Autodesk Inventor part; units mm, degrees
note: some values were not read from the file. Chosen so that the rebuilt part matches the saved one: direction of "Hole2".
(part 19 of 20)
  line L1608 (7.786286, -8.278547) -> (8.03493, -8.252551)
  line L1609 (8.03493, -8.252551) -> (8.035159, -8.252627)
  line L1610 (6.791707, -8.382529) -> (6.77091, -8.183613)
  line L1611 (6.543062, -8.408524) -> (6.791707, -8.382529)
  line L1612 (8.217517, -9.99687) -> (8.035159, -8.252627)
  line L1613 (7.010297, -10.471221) -> (7.274453, -10.443604)
  line L1614 (7.765489, -8.079631) -> (6.77091, -8.183613)
  line L1615 (6.543062, -8.408524) -> (6.740628, -10.298225)
  line L1616 (7.010069, -10.471145) -> (8.004648, -10.367163)
  line L1617 (8.232497, -10.142252) -> (8.03493, -8.252551)
  line L1618 (6.740856, -10.298301) -> (6.989283, -10.272328)
  line L1619 (6.740628, -10.298225) -> (6.740856, -10.298301)
  line L1620 (6.989273, -10.272229) -> (6.740628, -10.298225)
  line L1621 (7.010069, -10.471145) -> (6.989273, -10.272229)
  line L1622 (7.010297, -10.471221) -> (7.010069, -10.471145)
  line L1623 (7.983852, -10.168247) -> (8.004648, -10.367163)
  line L1624 (8.232497, -10.142252) -> (7.983852, -10.168247)
  line L1625 (6.812503, -8.581445) -> (6.968476, -10.073313)
  line L1626 (7.807082, -8.477462) -> (6.812503, -8.581445)
  line L1627 (7.963055, -9.969331) -> (7.807082, -8.477462)
  line L1628 (6.968476, -10.073313) -> (7.963055, -9.969331)
  line L1629 (7.125675, -9.879662) -> (7.006372, -8.738535)
  line L1630 (6.812503, -8.581445) -> (7.006372, -8.738535)
  line L1631 (6.968476, -10.073313) -> (7.125675, -9.879662)
  line L1632 (7.006372, -8.738535) -> (7.650209, -8.671223)
  line L1633 (7.807082, -8.477462) -> (7.650209, -8.671223)
  line L1634 (7.650209, -8.671223) -> (7.769512, -9.812349)
  line L1635 (7.963055, -9.969331) -> (7.769512, -9.812349)
  line L1636 (7.769512, -9.812349) -> (7.125675, -9.879662)
  circle A34 centre (7.360667, -9.014937) radius 0.1
  line L1637 (7.526698, -9.160376) -> (7.493026, -8.838309)
  line L1638 (7.526731, -9.160387) -> (7.526698, -9.160376)
  line L1639 (7.526731, -9.160387) -> (7.493059, -8.83832)
  line L1640 (7.493059, -8.83832) -> (7.493026, -8.838309)
  line L1641 (7.493026, -8.838309) -> (7.194653, -8.869503)
  line L1642 (7.194653, -8.869503) -> (7.228324, -9.191571)
  line L1643 (7.228357, -9.191582) -> (7.228324, -9.191571)
  line L1644 (7.228324, -9.191571) -> (7.526698, -9.160376)
  line L1645 (7.228357, -9.191582) -> (7.526731, -9.160387)
  line L1646 (3.439822, -8.704549) -> (3.439807, -8.9032)
  line L1647 (3.439807, -8.9032) -> (3.689807, -8.903219)
  line L1648 (2.439807, -8.903124) -> (2.439822, -8.704473)
  line L1649 (2.189807, -8.903105) -> (2.439807, -8.903124)
  line L1650 (3.439651, -10.952678) -> (3.689651, -10.952697)
  line L1651 (3.439664, -10.790392) -> (3.439648, -10.989044)
  line L1652 (3.689664, -10.790411) -> (3.439664, -10.790392)
  line L1653 (3.439648, -10.989044) -> (3.439636, -11.151329)
  line L1654 (3.689651, -10.952697) -> (3.689664, -10.790411)
  line L1655 (2.439636, -11.151253) -> (3.439636, -11.151329)
  line L1656 (3.439822, -8.704549) -> (2.439822, -8.704473)
  line L1657 (2.189807, -8.903105) -> (2.189664, -10.790297)
  line L1658 (2.439648, -10.988968) -> (3.439648, -10.989044)
  line L1659 (3.689664, -10.790411) -> (3.689807, -8.903219)
  line L1660 (2.189651, -10.952583) -> (2.439651, -10.952602)
  line L1661 (2.189664, -10.790297) -> (2.189651, -10.952583)
  line L1662 (2.439664, -10.790316) -> (2.189664, -10.790297)
  line L1663 (2.439648, -10.988968) -> (2.439664, -10.790316)
  line L1664 (2.439636, -11.151253) -> (2.439648, -10.988968)
  line L1665 (2.439792, -9.101776) -> (2.439679, -10.591664)
  line L1666 (3.439792, -9.101852) -> (2.439792, -9.101776)
  line L1667 (3.439679, -10.59174) -> (3.439792, -9.101852)
  line L1668 (2.439679, -10.591664) -> (3.439679, -10.59174)
  line L1669 (2.61601, -10.532458) -> (2.616097, -9.392846)
  line L1670 (2.439792, -9.101776) -> (2.616097, -9.392846)
  line L1671 (2.439679, -10.591664) -> (2.61601, -10.532458)
  line L1672 (2.616097, -9.392846) -> (3.263443, -9.392895)
  line L1673 (3.439792, -9.101852) -> (3.263443, -9.392895)
  line L1674 (3.263443, -9.392895) -> (3.263356, -10.532507)
  line L1675 (3.439679, -10.59174) -> (3.263356, -10.532507)
  line L1676 (3.263356, -10.532507) -> (2.61601, -10.532458)
  ellipse E661 centre (2.939748, -9.673551) end of major axis (2.839748, -9.673543) minor radius 0.099326
  ellipse E662 centre (2.939748, -9.679347) end of major axis (2.839748, -9.679339) minor radius 0.099326 (2.839748, -9.679339) -> (3.039748, -9.679355) ccw
  line L1677 (3.039748, -9.673559) -> (3.039748, -9.679355)
  line L1678 (2.839748, -9.673543) -> (2.839748, -9.679339)
  line L1679 (3.089736, -9.840178) -> (3.08976, -9.518539)
  line L1680 (3.089734, -9.863362) -> (3.089736, -9.840178)
  line L1681 (3.08976, -9.518539) -> (2.78976, -9.518516)
  line L1682 (2.78976, -9.518516) -> (2.789736, -9.840155)
  line L1683 (2.789734, -9.863339) -> (2.789736, -9.840155)
  line L1684 (2.789736, -9.840155) -> (3.089736, -9.840178)
  line L1685 (2.789734, -9.863339) -> (3.089734, -9.863362)
  line L1686 (8.477385, -9.966599) -> (8.477243, -9.966545)
  line L1687 (8.477243, -9.966545) -> (8.500438, -10.165195)
  line L1688 (8.500438, -10.165195) -> (8.748751, -10.136202)
  line L1689 (8.748751, -10.136202) -> (8.748892, -10.136257)
  line L1690 (8.969239, -12.023437) -> (8.748892, -10.136257)
  line L1691 (8.716449, -12.254311) -> (8.74412, -12.25108)
  line L1692 (8.477243, -9.966545) -> (8.2173, -9.996896)
  line L1693 (7.274441, -10.443505) -> (7.479218, -12.19734)
  line L1694 (7.750726, -12.366997) -> (8.743978, -12.251025)
  line L1695 (8.969097, -12.023382) -> (8.748751, -10.136202)
  line L1696 (8.7488, -12.049175) -> (8.969239, -12.023437)
  line L1697 (8.74412, -12.25108) -> (8.732832, -12.154407)
  line L1698 (8.720784, -12.052375) -> (8.743978, -12.251025)
  line L1699 (8.969097, -12.023382) -> (8.720784, -12.052375)
  line L1700 (8.720784, -12.052375) -> (8.720925, -12.052429)
  line L1701 (8.743978, -12.251025) -> (8.74412, -12.25108)
  line L1702 (8.969239, -12.023437) -> (8.969097, -12.023382)
  line L1703 (7.479218, -12.19734) -> (7.47936, -12.197394)
  line L1704 (7.727531, -12.168347) -> (7.479218, -12.19734)
  line L1705 (7.750726, -12.366997) -> (7.727531, -12.168347)
  line L1706 (7.750867, -12.367052) -> (7.750726, -12.366997)
  line L1707 (7.530379, -10.479817) -> (7.704337, -11.969696)
  line L1708 (8.523632, -10.363846) -> (7.530379, -10.479817)
  line L1709 (8.69759, -11.853724) -> (8.523632, -10.363846)
  line L1710 (7.704337, -11.969696) -> (8.69759, -11.853724)
  line L1711 (7.859126, -11.774149) -> (7.726067, -10.634545)
  line L1712 (7.530379, -10.479817) -> (7.726067, -10.634545)
  line L1713 (7.704337, -11.969696) -> (7.859126, -11.774149)
  line L1714 (7.726067, -10.634545) -> (8.369045, -10.559471)
  line L1715 (8.523632, -10.363846) -> (8.369045, -10.559471)
  line L1716 (8.369045, -10.559471) -> (8.502104, -11.699075)
  line L1717 (8.69759, -11.853724) -> (8.502104, -11.699075)
  line L1718 (8.502104, -11.699075) -> (7.859126, -11.774149)
  circle A35 centre (8.083686, -10.906656) radius 0.1
  line L1719 (8.251456, -11.050081) -> (8.213902, -10.728443)
  line L1720 (8.251476, -11.050089) -> (8.251456, -11.050081)
  line L1721 (8.251476, -11.050089) -> (8.213922, -10.728451)
  line L1722 (8.213922, -10.728451) -> (8.213902, -10.728443)
  line L1723 (8.213902, -10.728443) -> (7.915926, -10.763235)
  line L1724 (7.915926, -10.763235) -> (7.95348, -11.084873)
  line L1725 (7.953501, -11.08488) -> (7.95348, -11.084873)
  line L1726 (7.95348, -11.084873) -> (8.251456, -11.050081)
  line L1727 (7.953501, -11.08488) -> (8.251476, -11.050089)
  line L1728 (3.440093, -5.140062) -> (3.440078, -5.339171)
  line L1729 (3.440078, -5.339171) -> (3.690078, -5.33919)
  line L1730 (2.440078, -5.339095) -> (2.440093, -5.139986)
  line L1731 (2.190078, -5.339076) -> (2.440078, -5.339095)
  line L1732 (3.440093, -5.140062) -> (2.440093, -5.139986)
  line L1733 (2.190078, -5.339076) -> (2.189941, -7.14516)
  line L1734 (3.689941, -7.145274) -> (3.690078, -5.33919)
  line L1735 (2.440063, -5.538203) -> (2.439956, -6.946265)
  line L1736 (3.440063, -5.538279) -> (2.440063, -5.538203)
  line L1737 (3.439956, -6.946341) -> (3.440063, -5.538279)
  line L1738 (2.616333, -6.288782) -> (2.616369, -5.808082)
  line L1739 (2.440063, -5.538203) -> (2.616369, -5.808082)
  line L1740 (2.616369, -5.808082) -> (3.263715, -5.808131)
  line L1741 (3.440063, -5.538279) -> (3.263715, -5.808131)
  line L1742 (3.263715, -5.808131) -> (3.263679, -6.288832)
  ellipse E663 centre (2.940021, -6.094897) end of major axis (2.840021, -6.09489) minor radius 0.099554
  ellipse E664 centre (2.94002, -6.099613) end of major axis (2.84002, -6.099606) minor radius 0.099554 (2.84002, -6.099606) -> (3.04002, -6.099621) ccw
  line L1743 (3.040021, -6.094905) -> (3.04002, -6.099621)
  line L1744 (2.840021, -6.09489) -> (2.84002, -6.099606)
  line L1745 (3.090008, -6.260814) -> (3.090033, -5.938435)
  line L1746 (3.090007, -6.279679) -> (3.090008, -6.260814)
  line L1747 (3.090033, -5.938435) -> (2.790033, -5.938413)
  line L1748 (2.790033, -5.938413) -> (2.790008, -6.260792)
  line L1749 (2.790007, -6.279657) -> (2.790008, -6.260792)
  line L1750 (2.790008, -6.260792) -> (3.090008, -6.260814)
  line L1751 (2.790007, -6.279657) -> (3.090007, -6.279679)
  line L1752 (7.201687, -6.366416) -> (7.182831, -6.167323)
  line L1753 (7.182831, -6.167323) -> (7.182731, -6.167316)
  line L1754 (7.182731, -6.167316) -> (7.201589, -6.366425)
  line L1755 (7.201589, -6.366425) -> (7.450475, -6.342853)
  line L1756 (7.450475, -6.342853) -> (7.450575, -6.34286)
  line L1757 (6.206044, -6.460713) -> (6.187186, -6.261604)
  line L1758 (5.957157, -6.484285) -> (6.206044, -6.460713)
  line L1759 (7.471423, -6.562983) -> (7.450575, -6.34286)
  line L1760 (7.182731, -6.167316) -> (6.187186, -6.261604)
  line L1761 (5.957157, -6.484285) -> (6.136303, -8.37582)
  line L1762 (6.404047, -8.551357) -> (6.556485, -8.53692)
  line L1763 (7.61644, -8.095214) -> (7.450475, -6.342853)
  line L1764 (6.136303, -8.37582) -> (6.136404, -8.375826)
  line L1765 (6.38519, -8.352248) -> (6.136303, -8.37582)
  line L1766 (6.404047, -8.551357) -> (6.38519, -8.352248)
  line L1767 (6.404147, -8.551364) -> (6.404047, -8.551357)
  line L1768 (6.224901, -6.659822) -> (6.366332, -8.153139)
  line L1769 (7.220446, -6.565534) -> (6.224901, -6.659822)
  line L1770 (7.361877, -8.058852) -> (7.220446, -6.565534)
  line L1771 (6.366332, -8.153139) -> (7.361877, -8.058852)
  line L1772 (6.52532, -7.960977) -> (6.41714, -6.818742)
  line L1773 (6.224901, -6.659822) -> (6.41714, -6.818742)
  line L1774 (6.366332, -8.153139) -> (6.52532, -7.960977)
  line L1775 (6.41714, -6.818742) -> (7.061602, -6.757706)
  line L1776 (7.220446, -6.565534) -> (7.061602, -6.757706)
  line L1777 (7.061602, -6.757706) -> (7.169782, -7.89994)
  line L1778 (7.361877, -8.058852) -> (7.169782, -7.89994)
  line L1779 (7.169782, -7.89994) -> (6.52532, -7.960977)
  circle A36 centre (6.768748, -7.098596) radius 0.1
  line L1780 (6.933349, -7.245643) -> (6.902817, -6.923263)
  line L1781 (6.933364, -7.245644) -> (6.902831, -6.923263)
  line L1782 (6.902817, -6.923263) -> (6.604154, -6.951549)
  line L1783 (6.604154, -6.951549) -> (6.634686, -7.273929)
  line L1784 (6.634686, -7.273929) -> (6.933349, -7.245643)
  ellipse E665 centre (-10.520754, -10.238556) end of major axis (-11.719228, -10.299056) minor radius 0.214474 (-9.764112, -10.035048) -> (-11.697324, -10.33696) ccw
  ellipse E666 centre (-10.510833, -10.435086) end of major axis (-11.509561, -10.485502) minor radius 0.178729 (-9.978797, -10.257642) -> (-11.297119, -10.583852) ccw
  line L1785 (-11.491308, -10.517089) -> (-11.697324, -10.33696)
  ellipse E667 centre (-10.510833, -10.435086) end of major axis (-11.259879, -10.472898) minor radius 0.134046 (-10.235366, -10.296818) -> (-11.050291, -10.554562) ccw
  line L1786 (-11.719228, -10.299056) -> (-11.762061, -9.450552)
  ellipse E668 centre (10.530165, -10.240157) end of major axis (11.72863, -10.300839) minor radius 0.214474 (11.70672, -10.33874) -> (9.773554, -10.036533) ccw
  ellipse E669 centre (10.520214, -10.436685) end of major axis (11.518935, -10.487253) minor radius 0.178729 (11.306477, -10.585571) -> (9.988205, -10.259161) ccw
  line L1787 (11.500677, -10.518837) -> (11.70672, -10.33874)
  ellipse E670 centre (10.520214, -10.436685) end of major axis (11.269255, -10.474611) minor radius 0.134046 (11.059654, -10.556244) -> (10.244768, -10.298376) ccw
  line L1788 (11.72863, -10.300839) -> (11.771592, -9.452341)
  ellipse E671 centre (0.005822, 4.447603) end of major axis (-0.560598, 4.447646) minor radius 0.563895 (0.374763, 4.019735) -> (-0.363184, 4.019791) ccw
  line L1789 (-0.107751, 4.840436) -> (0.290762, 4.741938)
  line L1790 (0.290762, 4.741938) -> (0.404336, 4.349105)
  line L1791 (0.404336, 4.349105) -> (0.142592, 4.078731)
  line L1792 (-0.108974, 4.111214) -> (-0.279118, 4.153268)
  line L1793 (-0.279118, 4.153268) -> (-0.392691, 4.546101)
  line L1794 (-0.392691, 4.546101) -> (-0.107751, 4.840436)
  line L1795 (0.290762, 4.741938) -> (0.290756, 4.652243)
  line L1796 (-0.107758, 4.751181) -> (-0.107751, 4.840436)
  spline S53 degree 3 poles (-11.59262, -40.37168) (-11.587874, -40.372306) (-11.577549, -40.373667) (-11.562894, -40.383311) (-11.548322, -40.397841) (-11.53396, -40.418162) (-11.520082, -40.443816) (-11.501451, -40.486582) (-11.485653, -40.535603) (-11.472041, -40.590104) (-11.458687, -40.654476) (-11.445359, -40.742787) (-11.436003, -40.854008) (-11.432673, -40.968592) (-11.436021, -41.083176) (-11.445393, -41.194396) (-11.458735, -41.282705) (-11.472098, -41.347075) (-11.485719, -41.401574) (-11.501524, -41.450592) (-11.520162, -41.493356) (-11.534044, -41.519008) (-11.548409, -41.539326) (-11.562983, -41.553853) (-11.577639, -41.563495) (-11.587965, -41.564855) (-11.592711, -41.56548) knots 0 0 0 0 0.01106677 0.02407754 0.03992786 0.05913986 0.0819337 0.10802006 0.16805875 0.20201508 0.23929564 0.3216678 0.41056278 0.5 0.58943722 0.6783322 0.76070436 0.79798492 0.83194125 0.89197994 0.9180663 0.94086014 0.96007214 0.97592246 0.98893323 1 1 1 1
  spline S54 degree 3 poles (-11.592711, -41.56548) (-11.597373, -41.56487) (-11.60739, -41.56356) (-11.621305, -41.553879) (-11.634543, -41.539274) (-11.647072, -41.518918) (-11.658696, -41.49325) (-11.673818, -41.450356) (-11.685905, -41.401361) (-11.695951, -41.34698) (-11.705594, -41.28252) (-11.714843, -41.194166) (-11.721147, -41.083055) (-11.723326, -40.96857) (-11.72113, -40.854086) (-11.714809, -40.742975) (-11.705546, -40.654623) (-11.695894, -40.590164) (-11.68584, -40.535785) (-11.673744, -40.486792) (-11.658616, -40.4439) (-11.646989, -40.418234) (-11.634456, -40.39788) (-11.621216, -40.383277) (-11.607299, -40.373599) (-11.597282, -40.37229) (-11.59262, -40.37168) knots 0 0 0 0 0.01099744 0.02362844 0.03895388 0.0576141 0.07990846 0.10559498 0.1652091 0.19914929 0.2365432 0.31951534 0.40940333 0.5 0.59059667 0.68048466 0.7634568 0.80085071 0.8347909 0.89440502 0.92009154 0.9423859 0.96104612 0.97637156 0.98900256 1 1 1 1
  spline S55 degree 3 poles (11.597357, -41.567244) (11.592611, -41.566618) (11.582286, -41.565257) (11.56763, -41.555613) (11.553059, -41.541083) (11.538697, -41.520762) (11.524819, -41.495108) (11.506188, -41.452342) (11.49039, -41.403321) (11.476777, -41.34882) (11.463424, -41.284448) (11.450096, -41.196137) (11.44074, -41.084916) (11.43741, -40.970332) (11.440758, -40.855748) (11.45013, -40.744528) (11.463471, -40.656219) (11.476835, -40.591849) (11.490456, -40.53735) (11.506261, -40.488332) (11.524899, -40.445568) (11.538781, -40.419916) (11.553146, -40.399598) (11.567719, -40.385071) (11.582376, -40.375429) (11.592702, -40.374069) (11.597448, -40.373444) knots 0 0 0 0 0.01106677 0.02407754 0.03992786 0.05913986 0.0819337 0.10802006 0.16805875 0.20201508 0.23929564 0.3216678 0.41056278 0.5 0.58943722 0.6783322 0.76070436 0.79798492 0.83194125 0.89197994 0.9180663 0.94086014 0.96007214 0.97592246 0.98893323 1 1 1 1
  spline S56 degree 3 poles (11.597448, -40.373444) (11.60211, -40.374054) (11.612126, -40.375364) (11.626042, -40.385045) (11.63928, -40.39965) (11.651809, -40.420006) (11.663433, -40.445674) (11.678555, -40.488568) (11.690642, -40.537563) (11.700688, -40.591944) (11.71033, -40.656404) (11.71958, -40.744758) (11.725884, -40.855869) (11.728063, -40.970354) (11.725866, -41.084838) (11.719545, -41.195949) (11.710283, -41.284301) (11.700631, -41.34876) (11.690576, -41.403139) (11.678481, -41.452132) (11.663353, -41.495024) (11.651725, -41.52069) (11.639193, -41.541044) (11.625953, -41.555647) (11.612036, -41.565325) (11.602019, -41.566634) (11.597357, -41.567244) knots 0 0 0 0 0.01099744 0.02362844 0.03895388 0.0576141 0.07990846 0.10559498 0.1652091 0.19914929 0.2365432 0.31951534 0.40940333 0.5 0.59059667 0.68048466 0.7634568 0.80085071 0.8347909 0.89440502 0.92009154 0.9423859 0.96104612 0.97637156 0.98900256 1 1 1 1
  line L1797 (-4.211059, -43.377142) -> (-4.211066, -43.469142)
  line L1798 (-9.152053, -43.468766) -> (-9.152007, -42.868766)
  line L1799 (-4.211066, -43.469142) -> (-9.152053, -43.468766)
  line L1800 (4.215423, -43.469782) -> (4.21543, -43.377782)
  line L1801 (9.156409, -43.470158) -> (4.215423, -43.469782)
  line L1802 (9.156455, -42.870158) -> (9.156409, -43.470158)
  line L1803 (-3.997776, -42.869158) -> (-9.152007, -42.868766)
  line L1804 (9.156455, -42.870158) -> (4.002224, -42.869766)
  line L1805 (11.952178, -43.470371) -> (9.156409, -43.470158)
  line L1806 (-9.152053, -43.468766) -> (-11.947822, -43.468553)
  line L1807 (4.002559, -38.469766) -> (11.952559, -38.470371)
  line L1808 (-11.947441, -38.468553) -> (-3.997441, -38.469158)
  line L1809 (-11.947822, -43.468553) -> (-11.947441, -38.468553)
  line L1810 (11.952178, -43.470371) -> (11.952559, -38.470371)
  line L1811 (4.215423, -43.469782) -> (3.905563, -43.469759)
  line L1812 (3.905563, -43.469759) -> (3.90557, -43.377759)
  line L1813 (3.905563, -43.469759) -> (-4.211066, -43.469142)
  line L1814 (-9.079045, -28.468771) -> (-3.321818, -28.469209)
  line L1815 (3.328456, -28.469715) -> (9.085683, -28.470153)
  line L1816 (10.653551, -28.470272) -> (11.216615, -28.470315)
  line L1817 (-11.209977, -28.468609) -> (-10.646913, -28.468652)
  line L1818 (11.215854, -38.470315) -> (11.216615, -28.470315)
  line L1819 (-11.209977, -28.468609) -> (-11.210737, -38.468609)
  spline S57 degree 3 poles (-8.765036, -35.867834) (-8.764769, -35.757599) (-8.761349, -35.533673) (-8.743222, -35.201238) (-8.713054, -34.928041) (-8.679705, -34.738723) (-8.645211, -34.64651) (-8.621798, -34.584045) (-8.572571, -34.581581) (-8.544972, -34.621627) (-8.510145, -34.702211) (-8.473031, -34.888434) (-8.44157, -35.161759) (-8.42366, -35.493232) (-8.419288, -35.826558) (-8.426873, -36.159477) (-8.446891, -36.493359) (-8.478808, -36.765397) (-8.514628, -36.955068) (-8.547047, -37.046324) (-8.57088, -37.112013) (-8.620232, -37.11221) (-8.646582, -37.070723) (-8.67735, -36.990083) (-8.714426, -36.804321) (-8.743636, -36.531889) (-8.761168, -36.199722) (-8.765301, -35.977117) (-8.765036, -35.867834) knots 0 0 0 0 0.06370705 0.12949472 0.19191208 0.22368799 0.2382902 0.25135028 0.25660425 0.26301775 0.27714857 0.30853838 0.37103998 0.43687849 0.50002298 0.56369496 0.62938323 0.69283553 0.72316052 0.73857311 0.75180992 0.75696152 0.7632602 0.77795176 0.80804313 0.87131401 0.93684349 1 1 1 1
  spline S58 degree 3 poles (-10.961204, -35.786075) (-10.960572, -35.563356) (-10.950183, -35.239504) (-10.950113, -34.843101) (-10.912349, -34.685004) (-10.92157, -34.591209) (-10.884933, -34.581169) (-10.874211, -34.661615) (-10.855678, -34.748938) (-10.840659, -34.969236) (-10.82721, -35.239057) (-10.81991, -35.572905) (-10.815873, -36.019318) (-10.831573, -36.452197) (-10.835133, -36.849308) (-10.874852, -37.008191) (-10.865551, -37.102751) (-10.902892, -37.113246) (-10.911506, -37.030807) (-10.929507, -36.943774) (-10.941719, -36.722668) (-10.957752, -36.345334) (-10.961836, -36.009053) (-10.961204, -35.786075) knots 0 0 0 0 0.13139199 0.19506211 0.22486648 0.236537 0.23877104 0.24363774 0.27264718 0.30298792 0.36807806 0.43503205 0.49911295 0.63103815 0.69471519 0.72474683 0.73665002 0.73889428 0.74387281 0.77307947 0.80345172 0.86845517 1 1 1 1
  spline S59 degree 3 poles (8.426688, -35.787549) (8.427022, -35.677218) (8.430095, -35.452601) (8.451958, -35.123731) (8.481432, -34.843077) (8.528867, -34.676495) (8.564967, -34.584637) (8.613971, -34.583373) (8.657301, -34.645523) (8.687787, -34.756551) (8.724589, -34.96873) (8.751757, -35.244846) (8.768138, -35.576173) (8.772309, -35.909457) (8.765265, -36.242834) (8.745686, -36.572028) (8.715121, -36.851569) (8.671368, -37.019168) (8.639129, -37.111061) (8.589647, -37.114782) (8.545979, -37.049233) (8.518251, -36.940131) (8.476898, -36.727728) (8.449753, -36.452792) (8.430699, -36.119621) (8.426358, -35.896767) (8.426688, -35.787549) knots 0 0 0 0 0.06377364 0.12947571 0.19191728 0.22251596 0.23572674 0.24098241 0.24712107 0.27642984 0.3084167 0.37100213 0.43691035 0.50001881 0.5637377 0.62924964 0.69193924 0.72212339 0.73538665 0.74053978 0.7469427 0.77702751 0.80721947 0.87118814 0.93686953 1 1 1 1
  line L1820 (9.085683, -28.470153) -> (10.653551, -28.470272)
  line L1821 (-10.646913, -28.468652) -> (-9.079045, -28.468771)
  spline S60 degree 3 poles (10.823981, -35.869324) (10.82469, -35.64542) (10.826632, -35.311386) (10.851011, -34.9324) (10.859679, -34.739412) (10.883274, -34.654106) (10.87675, -34.588309) (10.91413, -34.584971) (10.917546, -34.630294) (10.937011, -34.702577) (10.945793, -34.894313) (10.960284, -35.162958) (10.965785, -35.495284) (10.96758, -35.940764) (10.964119, -36.386459) (10.943062, -36.763358) (10.935643, -36.958091) (10.914064, -37.040444) (10.921591, -37.112085) (10.883957, -37.111227) (10.880857, -37.065642) (10.861355, -36.992736) (10.84984, -36.80192) (10.827243, -36.425919) (10.823277, -36.091835) (10.823981, -35.869324) knots 0 0 0 0 0.13209168 0.19547472 0.22735918 0.24158397 0.25296859 0.25518606 0.26025608 0.27356013 0.30485536 0.36824052 0.43535326 0.4998067 0.63172546 0.69607433 0.72644443 0.74148548 0.75299654 0.75519516 0.76033444 0.77439415 0.80449955 0.86873005 1 1 1 1
  line L1822 (4.003131, -30.939766) -> (2.003688, -23.619614)
  line L1823 (-1.996312, -23.61931) -> (-3.996869, -30.939158)
  line L1824 (4.002263, -42.361766) -> (4.003131, -30.939766)
  line L1825 (-3.997737, -42.361158) -> (-3.996869, -30.939158)
  line L1826 (2.003688, -23.619614) -> (-1.996312, -23.61931)
  line L1827 (4.002263, -42.361766) -> (4.002185, -43.377766)
  line L1828 (-3.997737, -42.361158) -> (-3.997815, -43.377158)
  line L1829 (4.002185, -43.377766) -> (-3.997815, -43.377158)
  line L1830 (-8.122783, -43.376844) -> (-8.297643, -43.376831)
  line L1831 (-8.122744, -42.868844) -> (-8.122783, -43.376844)
  line L1832 (-4.420375, -43.377126) -> (-8.122783, -43.376844)
  line L1833 (-4.420375, -43.377126) -> (-3.997815, -43.377158)
  line L1834 (4.002185, -43.377766) -> (4.424746, -43.377798)
  line L1835 (8.127153, -43.37808) -> (4.424746, -43.377798)
  line L1836 (8.127192, -42.87008) -> (8.127153, -43.37808)
  line L1837 (8.302013, -43.378093) -> (8.127153, -43.37808)
  line L1838 (-8.297604, -42.868831) -> (-8.297643, -43.376831)
  line L1839 (8.302052, -42.870093) -> (8.302013, -43.378093)
  line L1840 (-10.99805, -46.468625) -> (11.00195, -46.470299)
  line L1841 (-11.000559, -79.468625) -> (10.99944, -79.470298)
  line L1842 (-11.000559, -79.468625) -> (-10.99805, -46.468625)
  line L1843 (10.99944, -79.470298) -> (11.00195, -46.470299)
  line L1844 (-9.396535, -46.468747) -> (-9.396307, -43.468747)
  line L1845 (-7.296535, -46.468907) -> (-7.296307, -43.468907)
  line L1846 (-1.04805, -46.469382) -> (-1.047822, -43.469382)
  line L1847 (1.05195, -46.469542) -> (1.052178, -43.469542)
  line L1848 (7.300435, -46.470017) -> (7.300663, -43.470017)
  line L1849 (9.400435, -46.470177) -> (9.400663, -43.470177)
  spline S61 degree 3 poles (-9.494, -108.299265) (-9.352975, -108.712955) (-9.066555, -109.553156) (-8.690144, -110.85923) (-8.369211, -112.235424) (-8.131096, -113.648007) (-7.981225, -115.049157) (-7.905778, -116.397457) (-7.880518, -117.699949) (-7.880477, -118.554616) (-7.880457, -118.976908) knots 0 0 0 0 0.13110718 0.26627767 0.40758133 0.55482273 0.69573025 0.83010398 0.95981582 1.08650249 1.08650249 1.08650249 1.08650249
  spline S62 degree 3 poles (-11.494, -103.994777) (-11.494, -103.994565) (-11.494, -103.993719) (-11.494, -103.991816) (-11.494, -103.988647) (-11.494, -103.984218) (-11.494, -103.978533) (-11.494, -103.971598) (-11.494, -103.963419) (-11.494, -103.954002) (-11.494, -103.94335) (-11.494, -103.931473) (-11.494, -103.918383) (-11.494, -103.904098) (-11.494, -103.888638) (-11.494, -103.872014) (-11.494, -103.85424) (-11.494, -103.842008) (-11.494, -103.835703) knots 0 0 0 0 0.00398745 0.01595749 0.03589091 0.06374884 0.09949715 0.14310174 0.1945285 0.2537433 0.32071204 0.39540061 0.47774624 0.56757484 0.66479437 0.76932497 0.8810868 1 1 1 1
  spline S63 degree 3 poles (-11.494, -103.835703) (-11.340511, -104.219325) (-11.035906, -104.980636) (-10.360902, -106.465477) (-9.840536, -107.566226) (-9.494, -108.299265) knots 0 0 0 0 0.25334256 0.50276707 1 1 1 1
  spline S64 degree 3 poles (6.82, -107.936025) (6.670381, -108.362536) (6.366171, -109.229734) (5.960088, -110.578238) (5.61055, -112.002567) (5.349184, -113.466376) (5.184151, -114.918043) (5.101007, -116.312657) (5.073188, -117.658233) (5.073146, -118.540795) (5.073126, -118.976908) knots 0 0 0 0 0.13558682 0.27568002 0.42231514 0.57532331 0.7214304 0.86036495 0.99429907 1.12513191 1.12513191 1.12513191 1.12513191
  line L1850 (4.82, -103.423007) -> (4.82, -118.976908)
  line L1851 (5.073126, -118.976908) -> (4.82, -118.976908)
  line L1852 (4.82, -118.976908) -> (2.82, -118.976908)
  spline S65 degree 3 poles (2.82, -118.976908) (2.82, -118.094597) (2.82, -116.750133) (2.82, -114.921918) (2.82, -113.473903) (2.82, -112.013017) (2.82, -110.588504) (2.82, -109.238435) (2.82, -108.36339) (2.82, -107.935722) knots 0 0 0 0 0.26469338 0.4033392 0.54846434 0.69909791 0.84160494 0.97581833 1.10411856 1.10411856 1.10411856 1.10411856
  spline S66 degree 3 poles (2.82, -107.935722) (3.172761, -107.199483) (3.70314, -106.092544) (4.283845, -104.779597) (4.598396, -104.011823) (4.745841, -103.620051) (4.82, -103.423007) knots 0 0 0 0 0.49596798 0.74569065 0.8720938 1 1 1 1
  spline S67 degree 3 poles (4.82, -103.423007) (4.901571, -103.448017) (5.064256, -103.497897) (5.314289, -103.548517) (5.566412, -103.580101) (5.820068, -103.590515) (6.073642, -103.580133) (6.325869, -103.548566) (6.575833, -103.497986) (6.738529, -103.448123) (6.82, -103.423154) knots 0 0 0 0 0.12572609 0.25074567 0.37552827 0.50000542 0.62458391 0.74924522 0.87443269 1 1 1 1
  spline S68 degree 3 poles (6.82, -103.423154) (6.82, -103.812495) (6.82, -104.578201) (6.82, -106.082491) (6.82, -107.197441) (6.82, -107.936025) knots 0 0 0 0 0.25882001 0.5090148 1 1 1 1
  line L1853 (-9.494, -92.476908) -> (-9.494, -108.299265)
  line L1854 (-9.494, -92.476908) -> (-7.494, -92.476908)
  line L1855 (-7.494, -92.476908) -> (-7.494, -118.976908)
  line L1856 (-11.494, -92.476908) -> (-11.494, -103.835703)
  line L1857 (-11.494, -92.476908) -> (-9.494, -92.476908)
  line L1858 (2.82, -92.476908) -> (2.82, -107.935722)
  line L1859 (2.82, -92.476908) -> (4.82, -92.476908)
  line L1860 (4.82, -92.476908) -> (4.82, -103.423007)
  line L1861 (4.82, -92.476908) -> (6.82, -92.476908)
  line L1862 (6.82, -92.476908) -> (6.82, -103.423154)
  line L1863 (2.074, -92.476908) -> (2.074, -118.976908)
  line L1864 (2.074, -92.476908) -> (2.82, -92.476908)
  line L1865 (4.074, -92.476908) -> (4.074, -118.976908)
  line L1866 (6.074, -92.476908) -> (6.074, -108.443836)
  spline S69 degree 3 poles (4.452757, -118.976908) (4.452776, -118.560328) (4.452815, -117.717405) (4.478204, -116.432917) (4.55406, -115.103328) (4.704762, -113.721214) (4.944183, -112.327247) (5.266658, -110.968902) (5.644655, -109.680138) (5.93238, -108.851632) (6.074, -108.443836) knots 0 0 0 0 0.12497306 0.25287553 0.38537145 0.52436553 0.66974205 0.80937847 0.9429718 1.07246485 1.07246485 1.07246485 1.07246485
  spline S70 degree 3 poles (6.074, -103.679656) (5.987844, -103.685166) (5.815633, -103.696178) (5.556559, -103.685271) (5.299044, -103.654389) (5.044108, -103.602056) (4.79294, -103.529684) (4.546775, -103.437786) (4.305741, -103.328881) (4.151428, -103.242796) (4.074, -103.199602) knots 0 0 0 0 0.12386032 0.2475762 0.37158497 0.495852 0.6207493 0.74643209 0.87276965 1 1 1 1
  spline S71 degree 3 poles (4.074, -103.199602) (4.001933, -103.38556) (3.858487, -103.755699) (3.550686, -104.481454) (3.141244, -105.369914) (2.617557, -106.417283) (2.255355, -107.107627) (2.074, -107.453285) knots 0 0 0 0 0.12719878 0.25318248 0.50275428 0.75102731 1 1 1 1
  line L1867 (12, -89.976908) -> (-12, -89.976908)
  line L1868 (9.484, 23.984) -> (-9.484, 23.984)
  line L1869 (9.970682, 23.598634) -> (-9.970682, 23.598634)
  spline S72 degree 3 poles (-10.984, 5) (-10.838244, 5.199129) (-10.544288, 5.600725) (-9.896796, 6.374089) (-9.217709, 7.133363) (-8.571526, 7.929913) (-8.202206, 8.45875) (-7.940907, 8.905409) (-7.76485, 9.255249) (-7.608484, 9.619751) (-7.525729, 9.872534) (-7.484, 10) knots 0 0 0 0 0.07401284 0.14926686 0.30244691 0.37959616 0.45685507 0.49566205 0.53474567 0.5742877 0.61450742 0.61450742 0.61450742 0.61450742
  spline S73 degree 3 poles (10.984, 5) (10.838244, 5.199129) (10.544288, 5.600725) (9.896796, 6.374089) (9.217709, 7.133363) (8.571526, 7.929913) (8.202206, 8.45875) (7.940907, 8.905409) (7.76485, 9.255249) (7.608484, 9.619751) (7.525729, 9.872534) (7.484, 10) knots 0 0 0 0 0.07401284 0.14926686 0.30244691 0.37959616 0.45685507 0.49566205 0.53474567 0.5742877 0.61450742 0.61450742 0.61450742 0.61450742
  spline S74 degree 3 poles (-12.5, 0) (-12.496854, 0.222811) (-12.490566, 0.668156) (-12.431105, 1.33272) (-12.325549, 1.988634) (-12.166009, 2.630572) (-11.95144, 3.254941) (-11.680705, 3.858812) (-11.359701, 4.443773) (-11.109771, 4.813796) (-10.984, 5) knots 0 0 0 0 0.06683217 0.13358148 0.19996019 0.26595386 0.33177154 0.39774949 0.46426825 0.53165054 0.53165054 0.53165054 0.53165054
  spline S75 degree 3 poles (12.5, 0) (12.496854, 0.222811) (12.490566, 0.668156) (12.431105, 1.33272) (12.325549, 1.988634) (12.166009, 2.630572) (11.95144, 3.254941) (11.680705, 3.858812) (11.359701, 4.443773) (11.109771, 4.813796) (10.984, 5) knots 0 0 0 0 0.06683217 0.13358148 0.19996019 0.26595386 0.33177154 0.39774949 0.46426825 0.53165054 0.53165054 0.53165054 0.53165054
  arc A37 (9.970682, 23.598634) -> (9.484, 23.984) centre (9.484, 23.484) ccw
  arc A38 (-9.484, 23.984) -> (-9.970682, 23.598634) centre (-9.484, 23.484) ccw
  spline S76 degree 3 poles (-7.484, 10) (-7.429867, 10.200851) (-7.319048, 10.612023) (-7.234695, 11.26385) (-7.207256, 11.956347) (-7.244824, 12.691551) (-7.341158, 13.468092) (-7.492838, 14.284777) (-7.695796, 15.138652) (-8.029407, 16.344887) (-8.525501, 17.903065) (-9.149713, 19.799331) (-9.609092, 21.401876) (-9.877301, 22.670977) (-9.94005, 23.294328) (-9.970682, 23.598634) knots 0 0 0 0 0.06234657 0.1276327 0.1966407 0.27004939 0.34820305 0.43123424 0.51911498 0.61142292 0.80662861 1.00959387 1.21035176 1.30648489 1.39817641 1.39817641 1.39817641 1.39817641
  spline S77 degree 3 poles (7.484, 10) (7.429867, 10.200851) (7.319048, 10.612023) (7.234695, 11.26385) (7.207256, 11.956347) (7.244824, 12.691551) (7.341158, 13.468092) (7.492838, 14.284777) (7.695796, 15.138652) (8.029407, 16.344887) (8.525501, 17.903065) (9.149713, 19.799331) (9.609092, 21.401876) (9.877301, 22.670977) (9.94005, 23.294328) (9.970682, 23.598634) knots 0 0 0 0 0.06234657 0.1276327 0.1966407 0.27004939 0.34820305 0.43123424 0.51911498 0.61142292 0.80662861 1.00959387 1.21035176 1.30648489 1.39817641 1.39817641 1.39817641 1.39817641
  line L1870 (11, 25) -> (-11, 25)
  spline S78 degree 3 poles (-8.5, 10) (-8.600541, 9.783932) (-8.803777, 9.347164) (-9.178711, 8.717278) (-9.586827, 8.086011) (-10.027701, 7.453058) (-10.497433, 6.823494) (-11.158647, 6.006378) (-11.664247, 5.401609) (-12, 5) knots 0 0 0 0 0.07145122 0.1444341 0.21963753 0.29697342 0.37578786 0.45523025 0.61227239 0.61227239 0.61227239 0.61227239
  spline S79 degree 3 poles (8.5, 10) (8.600541, 9.783932) (8.803777, 9.347164) (9.178711, 8.717278) (9.586827, 8.086011) (10.027701, 7.453058) (10.497433, 6.823494) (11.158647, 6.006378) (11.664247, 5.401609) (12, 5) knots 0 0 0 0 0.07145122 0.1444341 0.21963753 0.29697342 0.37578786 0.45523025 0.61227239 0.61227239 0.61227239 0.61227239
  spline S80 degree 3 poles (-12, 5) (-12.143547, 4.81536) (-12.357248, 4.540484) (-12.612885, 4.157085) (-12.786727, 3.86714) (-12.942184, 3.571631) (-13.078658, 3.270378) (-13.195004, 2.962903) (-13.291317, 2.649379) (-13.368568, 2.330191) (-13.447068, 1.896209) (-13.502651, 1.3423) (-13.519072, 0.672251) (-13.517023, 0.22399) (-13.516, 0) knots 0 0 0 0 0.07013118 0.1044054 0.13817293 0.17150982 0.2045203 0.23732848 0.27006639 0.30285264 0.33579 0.40230943 0.46959172 0.53678969 0.53678969 0.53678969 0.53678969
  spline S81 degree 3 poles (12, 5) (12.143547, 4.81536) (12.357248, 4.540484) (12.612885, 4.157085) (12.786727, 3.86714) (12.942184, 3.571631) (13.078658, 3.270378) (13.195004, 2.962903) (13.291317, 2.649379) (13.368568, 2.330191) (13.447068, 1.896209) (13.502651, 1.3423) (13.519072, 0.672251) (13.517023, 0.22399) (13.516, 0) knots 0 0 0 0 0.07013118 0.1044054 0.13817293 0.17150982 0.2045203 0.23732848 0.27006639 0.30285264 0.33579 0.40230943 0.46959172 0.53678969 0.53678969 0.53678969 0.53678969
  spline S82 degree 3 poles (-11, 23.984) (-10.983157, 23.66696) (-10.947704, 22.99964) (-10.734931, 21.978031) (-10.455281, 20.904433) (-10.004632, 19.44227) (-9.511797, 18.000831) (-9.042024, 16.593046) (-8.729519, 15.605995) (-8.467906, 14.680109) (-8.2663, 13.821987) (-8.130123, 13.034093) (-8.066603, 12.314867) (-8.076482, 11.660229) (-8.155308, 11.062944) (-8.295662, 10.511618) (-8.432528, 10.168935) (-8.5, 10) knots 0 0 0 0 0.09512154 0.200216 0.31218274 0.42803367 0.65906444 0.76919754 0.87325746 0.96964043 1.05776849 1.13759246 1.20931346 1.27406394 1.33359113 1.38967504 1.44420495 1.44420495 1.44420495 1.44420495
  spline S83 degree 3 poles (11, 23.984) (10.983157, 23.66696) (10.947704, 22.99964) (10.734931, 21.978031) (10.455281, 20.904433) (10.004632, 19.44227) (9.511797, 18.000831) (9.042024, 16.593046) (8.729519, 15.605995) (8.467906, 14.680109) (8.2663, 13.821987) (8.130123, 13.034093) (8.066603, 12.314867) (8.076482, 11.660229) (8.155308, 11.062944) (8.295662, 10.511618) (8.432528, 10.168935) (8.5, 10) knots 0 0 0 0 0.09512154 0.200216 0.31218274 0.42803367 0.65906444 0.76919754 0.87325746 0.96964043 1.05776849 1.13759246 1.20931346 1.27406394 1.33359113 1.38967504 1.44420495 1.44420495 1.44420495 1.44420495
  line L1871 (-11, 23.984) -> (-11, 25)
  line L1872 (11, 23.984) -> (11, 25)
  line L1873 (8, -118.976908) -> (5.073126, -118.976908)
  line L1874 (2.82, -118.976908) -> (-7.880457, -118.976908)
  spline S84 degree 3 poles (-13.016, -93.976908) (-13.015207, -94.829167) (-13.014019, -96.105329) (-12.913213, -97.801334) (-12.774751, -99.062904) (-12.564663, -100.314439) (-12.278307, -101.55424) (-11.923071, -102.783611) (-11.637393, -103.590013) (-11.494, -103.994777) knots 0 0 0 0 0.25561003 0.38274706 0.50949551 0.6361782 0.76322409 0.89103186 1.01983443 1.01983443 1.01983443 1.01983443
  spline S85 degree 3 poles (13.016, -93.976908) (13.011455, -95.046927) (13.004652, -96.648649) (12.821153, -98.774131) (12.562626, -100.349343) (12.185656, -101.905584) (11.543448, -103.967206) (10.508, -106.476908) (9.472552, -108.98661) (8.830344, -111.048232) (8.453374, -112.604472) (8.194847, -114.179685) (8.011348, -116.305167) (8.004545, -117.906889) (8, -118.976908) knots 0 0 0 0 0.32084871 0.48028147 0.63946219 0.79924314 0.96029185 1.28673686 1.61318187 1.77423059 1.93401153 2.09319225 2.25262502 2.57347372 2.57347372 2.57347372 2.57347372
  line L1875 (5, -89.976908) -> (5, -118.976908)
  line L1876 (-5, -89.976908) -> (-5, -118.976908)
  line L1877 (4.963, -89.976908) -> (4.963, -92.476908)
  line L1878 (3.185, -89.976908) -> (3.185, -92.476908)
  line L1879 (5.709, -89.976908) -> (5.709, -92.476908)
  line L1880 (3.931, -89.976908) -> (3.931, -92.476908)
  line L1881 (-8.605, -89.976908) -> (-8.605, -92.476908)
  line L1882 (-10.383, -89.976908) -> (-10.383, -92.476908)
  line L1883 (-12, -89.976908) -> (-12, -29.976908)
  line L1884 (12, -89.976908) -> (12, -29.976908)
  line L1885 (-13.016, -93.976908) -> (-13.016, -29.976908)
  line L1886 (13.016, -93.976908) -> (13.016, -29.976908)
  spline S86 degree 3 poles (-12, -29.976908) (-12.000338, -29.768116) (-12.001012, -29.35094) (-12.039011, -28.725642) (-12.125914, -28.104294) (-12.25, -27.488454) (-12.374086, -26.872614) (-12.460989, -26.251266) (-12.498988, -25.625968) (-12.499662, -25.208792) (-12.5, -25) knots 0 0 0 0 0.0626312 0.12513986 0.18776052 0.25067229 0.31358405 0.37620471 0.43871337 0.50134457 0.50134457 0.50134457 0.50134457
  spline S87 degree 3 poles (12, -29.976908) (12.000338, -29.768116) (12.001012, -29.35094) (12.039011, -28.725642) (12.125914, -28.104294) (12.25, -27.488454) (12.374086, -26.872614) (12.460989, -26.251266) (12.498988, -25.625968) (12.499662, -25.208792) (12.5, -25) knots 0 0 0 0 0.0626312 0.12513986 0.18776052 0.25067229 0.31358405 0.37620471 0.43871337 0.50134457 0.50134457 0.50134457 0.50134457
  spline S88 degree 3 poles (-13.516, -25) (-13.515662, -25.208792) (-13.514988, -25.625968) (-13.476989, -26.251266) (-13.390086, -26.872614) (-13.266, -27.488454) (-13.141914, -28.104294) (-13.055011, -28.725642) (-13.017012, -29.35094) (-13.016338, -29.768116) (-13.016, -29.976908) knots 0 0 0 0 0.0626312 0.12513986 0.18776052 0.25067229 0.31358405 0.37620471 0.43871337 0.50134457 0.50134457 0.50134457 0.50134457
  spline S89 degree 3 poles (13.516, -25) (13.515662, -25.208792) (13.514988, -25.625968) (13.476989, -26.251266) (13.390086, -26.872614) (13.266, -27.488454) (13.141914, -28.104294) (13.055011, -28.725642) (13.017012, -29.35094) (13.016338, -29.768116) (13.016, -29.976908) knots 0 0 0 0 0.0626312 0.12513986 0.18776052 0.25067229 0.31358405 0.37620471 0.43871337 0.50134457 0.50134457 0.50134457 0.50134457
  line L1887 (-12.5, -25) -> (-12.5, 0)
  line L1888 (12.5, -25) -> (12.5, 0)
  line L1889 (-13.516, -25) -> (-13.516, 0)
  line L1890 (13.516, -25) -> (13.516, 0)
  point P0 (0, 0)
  constraints: 4 end point, 1 parallel, 1 vertical, 2 other
sketch "Sketch14" plane through (0, 0, 0) normal (1, 0, 0) x (0, 1, 0)
  line L0 (-13.762, -15) -> (-13.762, 0)
  line L1 (13.762, 0) -> (-13.762, 0)
  line L2 (13.762, -15) -> (13.762, 0)
  line L3 (13, 0) -> (13, -15)
  line L4 (-13, 0) -> (-13, -15)
  line L5 (-13, 33) -> (6.5, 33)
  line L6 (6.5, 33) -> (6.5, 0)
  line L7 (6.5, 0) -> (-7.5, 0)
  line L8 (0, -156.78708) -> (0, 91.844197)
  line L9 (-6.5, 31.984) -> (6.5, 31.984)
  line L10 (-6.5, 31.984) -> (-6.5, 33)
  line L11 (-13.762, 0) -> (-13, 0)
  line L12 (0, 33) -> (0, 31.984)
  spline S0 degree 4 poles (-6.5, 31.984) (-9.3531, 31.984) (-16.854107, 30.644936) (-7.523287, 18.751181) (-11.13559, 10.231749) (-13, 3.906547) (-13, 0) knots 0 0 0 0 0 0.3528838 0.6028838 1 1 1 1 1
  spline S1 degree 4 poles (-6.5, 33) (-9.83171, 33) (-18.05171, 30.249728) (-8.631444, 19.983988) (-12.053674, 9.103926) (-13.762, 3.687137) (-13.762, 0) knots 0 0 0 0 0 0.36403398 0.61403398 1 1 1 1 1
  point P0 (0, 0)
  point P1 (0, 0)
  point P2 (-12.746, 29.495255)
  point P3 (-11.133597, 20.567754)
  point P4 (-11.133503, 10.338199)
  point P5 (-13.762, 29.495255)
  point P6 (-12.149597, 20.567806)
  point P7 (-12.149503, 9.405205)
  dimension "d94" = 33
  dimension "d95" = 1.016
  dimension "d96" = 13
  dimension "d203" = 1.016
  dimension "d204" = 1.016
  dimension "d205" = 1.016
  constraints: 14 end point, 5 point on line, 3 horizontal, 2 collinear, 2 midpoint, 2 parallel, 2 perpendicular, 2 vertical, 2 vertical alignment, 10 other
  measures "d94" distance between parallel lines of L1 L5
  measures "d95" distance between parallel lines of L9 L5
  measures "d96" distance between parallel lines of L6 L10
  measures "d203" distance of point (-12.746, 29.495) point (-13.762, 29.495)
  measures "d204" horizontal distance of point (-11.134, 10.338) point (-12.15, 9.405)
  measures "d205" distance of point (-11.134, 20.568) point (-12.15, 20.568)
revolve "Head" add sketch "Sketch14" angle 360 about axis through (0, 0, -10) along (0, 0, 1) contours L1 S1 L10 S0 | L10 L5 L8 L9
ref_plane "Work Plane8" through (0, 0, -109.976908) normal (0, 0, 1) x (1, 0, 0)
ref_plane "Work Plane9" through (0, 0, -83.976908) normal (0, 0, 1) x (1, 0, 0)
sketch "Sketch15" plane through (0, 0, -109.976908) normal (0, 0, 1) x (1, 0, 0)
  circle A0 centre (-8.737, 4.074) radius 0.889
  circle A1 centre (8.349, 4.82) radius 0.889
  circle A2 centre (0, -9.494) radius 0.889
  line L0 (-9.891701, 2.074) -> (-7.582299, 2.074)
  line L1 (-11.046401, 4.074) -> (-9.891701, 2.074)
  line L2 (-7.582299, 2.074) -> (-6.427599, 4.074)
  line L3 (-9.891701, 6.074) -> (-11.046401, 4.074)
  line L4 (-7.582299, 6.074) -> (-9.891701, 6.074)
  line L5 (-6.427599, 4.074) -> (-7.582299, 6.074)
  line L6 (1.154701, -7.494) -> (-1.154701, -7.494)
  line L7 (2.309401, -9.494) -> (1.154701, -7.494)
  line L8 (1.154701, -11.494) -> (2.309401, -9.494)
  line L9 (-1.154701, -11.494) -> (1.154701, -11.494)
  line L10 (-2.309401, -9.494) -> (-1.154701, -11.494)
  line L11 (-1.154701, -7.494) -> (-2.309401, -9.494)
  line L12 (7.194299, 6.82) -> (6.039599, 4.82)
  line L13 (9.503701, 6.82) -> (7.194299, 6.82)
  line L14 (10.658401, 4.82) -> (9.503701, 6.82)
  line L15 (9.503701, 2.82) -> (10.658401, 4.82)
  line L16 (7.194299, 2.82) -> (9.503701, 2.82)
  line L17 (6.039599, 4.82) -> (7.194299, 2.82)
  point P0 (0, 0)
  point P1 (0, 0)
  constraints: 36 end point, 3 centre point
hole "Hole3" at (0, -9.494, -109.976908) at (-8.737, 4.074, -109.976908) at (8.349, 4.82, -109.976908) direction (0, 0, 1) diameter 6 depth 26
ref_plane "Work Plane10" through (0, 13.762, -7.5) normal (0, 1, 0) x (-1, 0, 0)
sketch "Sketch16" plane through (0, 13.762, -7.5) normal (0, 1, 0) x (-1, 0, 0)
  line L0 (13.016, -22.476908) -> (-13.016, -22.476908)
  line L1 (-13.016, -76.476908) -> (-13.016, -22.476908)
  line L2 (0, -149.28708) -> (0, 99.344197)
  line L3 (0, -22.476908) -> (0, -7.5)
  line L4 (13.762, -7.5) -> (-13.762, -7.5)
  line L5 (13.016, -22.476908) -> (-13.016, -22.476908)
  line L6 (0, -7.5) -> (0, -22.476908)
  line L7 (0, -7.5) -> (0, 7.5)
  line L8 (-13.762, -7.5) -> (-13.762, 7.5)
  line L9 (13.762, -7.5) -> (13.762, 7.5)
  line L10 (-13, 7.5) -> (-13, -7.5)
  line L11 (13, 7.5) -> (13, -7.5)
  line L12 (13.762, 7.5) -> (-13.762, 7.5)
  line L13 (0, -7.5) -> (0, 7.5)
  line L14 (-19.2668, -72.476908) -> (19.2668, -72.476908)
  line L15 (6.5, 40.5) -> (-6.5, 40.5)
  line L16 (-11, 12.5) -> (11, 12.5)
  line L17 (11, 12.5) -> (11, 7.5)
  line L18 (11, 7.5) -> (-11, 7.5)
  line L19 (-11, 7.5) -> (-11, 12.5)
  line L20 (-11, 7.5) -> (11, 7.5)
  line L21 (11, 7.5) -> (11, -7.5)
  line L22 (11, -7.5) -> (-11, -7.5)
  line L23 (-11, -7.5) -> (-11, 7.5)
  line L24 (-11, -7.5) -> (11, -7.5)
  line L25 (11, -7.5) -> (11, -22.476908)
  line L26 (11, -22.476908) -> (-11, -22.476908)
  line L27 (-11, -22.476908) -> (-11, -7.5)
  line L28 (-11, -22.476908) -> (11, -22.476908)
  line L29 (11, -22.476908) -> (11, -32.476908)
  line L30 (11, -32.476908) -> (-11, -32.476908)
  line L31 (-11, -32.476908) -> (-11, -22.476908)
  line L32 (-9.984, 11.484) -> (9.984, 11.484)
  line L33 (9.984, 11.484) -> (9.984, 7.5)
  line L34 (9.984, 7.5) -> (-9.984, 7.5)
  line L35 (-9.984, 7.5) -> (-9.984, 11.484)
  line L36 (-9.984, 7.5) -> (9.984, 7.5)
  line L37 (9.984, 7.5) -> (9.984, -7.5)
  line L38 (9.984, -7.5) -> (-9.984, -7.5)
  line L39 (-9.984, -7.5) -> (-9.984, 7.5)
  line L40 (-9.984, -7.5) -> (9.984, -7.5)
  line L41 (9.984, -7.5) -> (9.984, -22.476908)
  line L42 (9.984, -22.476908) -> (-9.984, -22.476908)
  line L43 (-9.984, -22.476908) -> (-9.984, -7.5)
  line L44 (-9.984, -22.476908) -> (9.984, -22.476908)
  line L45 (8.976, -32.476908) -> (-8.976, -32.476908)
  line L46 (-9.984, -22.476908) -> (9.984, -22.476908)
  line L47 (9.984, -22.476908) -> (9.984, -31.460908)
  line L48 (9.984, -31.460908) -> (-9.984, -31.460908)
  line L49 (-9.984, -31.460908) -> (-9.984, -22.476908)
  arc A0 (3.065331, 35.369841) -> (3.065331, 35.369841) centre (3.065331, 35.369841) ccw
  arc A1 (3.065331, 35.369841) -> (3.065331, 35.369841) centre (3.065331, 35.369841) ccw
  point P0 (0, 40.5)
  point P1 (0, -7.5)
  point P2 (0, 12.5)
  point P3 (0, 7.5)
  point P4 (0, 7.5)
  point P5 (0, 7.5)
  point P6 (0, 11.484)
  dimension "d112" = 22
  dimension "d127" = 10
  dimension "d128" = 5
  dimension "d129" = 1.016
  dimension "d130" = 1.016
  dimension "d131" = 1.016
  constraints: 68 end point, 17 parallel, 9 horizontal, 8 coincident, 8 perpendicular, 8 point on line, 6 midpoint, 2 vertical alignment, 3 other
  measures "d112" distance between parallel lines of L17 L19
  measures "d127" distance between parallel lines of L30 L26
  measures "d128" distance between parallel lines of L18 L16
  measures "d129" distance between parallel lines of L35 L19
  measures "d130" distance between parallel lines of L45 L48
  measures "d131" distance between parallel lines of L32 L16
extrude "Extrusion4" [suppressed]
sketch "Sketch16 outline for Extrusion8" plane through (0, 13.762, -7.5) normal (0, 1, 0) x (-1, 0, 0)
  line L0 (11, 7.5) -> (-11, 7.5)
  line L1 (11, -7.5) -> (11, 7.5)
  line L2 (-11, -7.5) -> (11, -7.5)
  line L3 (-11, 7.5) -> (-11, -7.5)
extrude "Extrusion8" add sketch "Sketch16 outline for Extrusion8" against normal up to surface
sketch "Sketch16 outline for Extrusion6" plane through (0, 13.762, -7.5) normal (0, 1, 0) x (-1, 0, 0)
  line L0 (11, -7.5) -> (-11, -7.5)
  line L1 (11, -22.476908) -> (11, -7.5)
  line L2 (-11, -22.476908) -> (11, -22.476908)
  line L3 (-11, -7.5) -> (-11, -22.476908)
extrude "Extrusion6" add sketch "Sketch16 outline for Extrusion6" against normal up to next
sketch "Sketch16 outline for Extrusion7" plane through (0, 13.762, -7.5) normal (0, 1, 0) x (-1, 0, 0)
  line L0 (11, -22.476908) -> (-11, -22.476908)
  line L1 (11, -32.476908) -> (11, -22.476908)
  line L2 (-11, -32.476908) -> (11, -32.476908)
  line L3 (-11, -22.476908) -> (-11, -32.476908)
extrude "Extrusion7" add sketch "Sketch16 outline for Extrusion7" against normal up to surface
extrude "Extrusion9" [suppressed]
sketch "Sketch16 outline for Extrusion10" plane through (0, 13.762, -7.5) normal (0, 1, 0) x (-1, 0, 0)
  line L0 (-9.984, -7.5) -> (9.984, -7.5)
  line L1 (-9.984, 7.5) -> (-9.984, -7.5)
  line L2 (9.984, 7.5) -> (-9.984, 7.5)
  line L3 (9.984, -7.5) -> (9.984, 7.5)
extrude "Extrusion10" cut sketch "Sketch16 outline for Extrusion10" against normal up to surface
sketch "Sketch16 outline for Extrusion11" plane through (0, 13.762, -7.5) normal (0, 1, 0) x (-1, 0, 0)
  line L0 (-9.984, -22.476908) -> (9.984, -22.476908)
  line L1 (-9.984, -7.5) -> (-9.984, -22.476908)
  line L2 (9.984, -7.5) -> (-9.984, -7.5)
  line L3 (9.984, -22.476908) -> (9.984, -7.5)
extrude "Extrusion11" cut sketch "Sketch16 outline for Extrusion11" against normal blind 10
sketch "Sketch16 outline for Extrusion12" plane through (0, 13.762, -7.5) normal (0, 1, 0) x (-1, 0, 0)
  line L0 (9.984, -22.476908) -> (-9.984, -22.476908)
  line L1 (9.984, -31.460908) -> (9.984, -22.476908)
  line L2 (-9.984, -31.460908) -> (9.984, -31.460908)
  line L3 (-9.984, -22.476908) -> (-9.984, -31.460908)
extrude "Extrusion12" cut sketch "Sketch16 outline for Extrusion12" against normal up to surface
sketch "Sketch18" plane through (0, 13.762, -7.5) normal (0, 1, 0) x (1, 0, 0)
  line L0 (-9.984, -11.484) -> (-9.984, 31.460908)
  line L1 (-9.984, 31.460908) -> (9.984, 31.460908)
  line L2 (9.984, 31.460908) -> (9.984, -11.484)
  line L3 (9.984, -11.484) -> (-9.984, -11.484)
  line L4 (11, -12.5) -> (11, 32.476908)
  line L5 (11, 32.476908) -> (-11, 32.476908)
  line L6 (-11, 32.476908) -> (-11, -12.5)
  line L7 (-11, -12.5) -> (11, -12.5)
  point P0 (0, -7.5)
extrude "Extrusion13" [suppressed]
sketch "Sketch19" plane through (0, 25.262, -7.5) normal (0, 1, 0) x (1, 0, 0)
  line L0 (-10.684699, 31.685607) -> (10.579594, 31.685607)
  line L1 (10.579594, 31.685607) -> (10.579594, -12.184699)
  line L2 (10.579594, -12.184699) -> (-10.684699, -12.184699)
  line L3 (-10.684699, -12.184699) -> (-10.684699, 31.685607)
  line L4 (-12.208699, 33.685607) -> (12.208699, 33.685607)
  line L5 (12.208699, -13.708699) -> (-12.208699, -13.708699)
  line L6 (-12.208699, -13.708699) -> (-12.208699, 33.685607)
  point P0 (0, -7.5)
  point P1 (-0.052552, 31.685607)
  point P2 (-0.052552, 30.813551)
  dimension "d183" = 2
  dimension "d184" = 1.524
  dimension "d185" = 1.524
  constraints: 8 end point, 2 parallel, 1 horizontal, 1 midpoint, 1 perpendicular, 1 vertical alignment
  measures "d183" distance between parallel lines of L0 L4
  measures "d184" distance between parallel lines of L5 L2
  measures "d185" distance between parallel lines of L3 L6